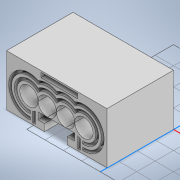
# Autodesk Inventor part: Part1
Saved by Autodesk Inventor 2020.3 (Build 243373010, 373A)
## iProperties
Created: 2021-11-04
Part Number: Part1
Material: Generic
Document SubType Name: Modeling
Designer: joesp
Density: 1 g/cm^3
Appearance: Default
Author: joesp
Autodesk Inventor part; units mm, degrees
ref_plane "YZ Plane" through (0, 0, 0) normal (1, 0, 0) x (0, 1, 0)
ref_plane "XZ Plane" through (0, 0, 0) normal (0, 1, 0) x (-1, 0, 0)
ref_plane "XY Plane" through (0, 0, 0) normal (0, 0, 1) x (1, 0, 0)
sketch "Sketch2" plane through (0, 0, 0) normal (0, 0, 1) x (1, 0, 0)
  line L0 (0, 0) -> (-109.5178, 0)
  line L1 (-109.5178, 0) -> (-109.5178, 55.7873)
  line L2 (-109.5178, 55.7873) -> (0, 55.7873)
  line L3 (0, 55.7873) -> (0, 0)
  circle A0 centre (-85.0707, 25.2343) radius 10
  circle A1 centre (-65.0707, 25.2343) radius 10
  circle A2 centre (-45.0707, 25.2343) radius 10
  circle A3 centre (-25.0707, 25.2343) radius 10
  line L4 (-71.9158, 54.2) -> (-31.9158, 54.2)
  line L5 (-31.9158, 54.2) -> (-31.9158, 49.2)
  line L6 (-31.9158, 49.2) -> (-71.9158, 49.2)
  line L7 (-71.9158, 49.2) -> (-71.9158, 54.2)
  line L8 (-68.1085, 0) -> (-68.1085, 7.7343)
  line L9 (-68.1085, 7.7343) -> (-75.0707, 7.7343)
  line L10 (-75.0707, 7.7343) -> (-75.0707, 15.2343)
  line L11 (-75.0707, 15.2343) -> (-35.0707, 15.2343)
  line L12 (-35.0707, 15.2343) -> (-35.0707, 7.7343)
  line L13 (-35.0707, 7.7343) -> (-43.2815, 7.7343)
  line L14 (-43.2815, 7.7343) -> (-43.2815, 0)
  arc A4 (-75.0707, 33.5409) -> (-76.764, 15.2343) centre (-85.0707, 25.2343) ccw
  arc A5 (-55.0707, 33.5409) -> (-75.0707, 33.5409) centre (-65.0707, 25.2343) ccw
  arc A6 (-35.0707, 33.5409) -> (-55.0707, 33.5409) centre (-45.0707, 25.2343) ccw
  arc A7 (-33.3773, 15.2343) -> (-35.0707, 33.5409) centre (-25.0707, 25.2343) ccw
  line L15 (-76.764, 15.2343) -> (-75.0707, 15.2343)
  line L16 (-33.3773, 15.2343) -> (-35.0707, 15.2343)
  arc A8 (-75.0707, 37.7243) -> (-81.0707, 9.7424) centre (-85.0707, 25.2343) ccw
  arc A9 (-55.0707, 37.7243) -> (-75.0707, 37.7243) centre (-65.0707, 25.2343) ccw
  arc A10 (-35.0707, 37.7243) -> (-55.0707, 37.7243) centre (-45.0707, 25.2343) ccw
  arc A11 (-29.0707, 9.7424) -> (-35.0707, 37.7243) centre (-25.0707, 25.2343) ccw
  line L17 (-78.0707, 2) -> (-81.0707, 2)
  line L18 (-81.0707, 2) -> (-81.0707, 14.2799)
  line L19 (-81.0707, 14.2799) -> (-78.0707, 14.2799)
  line L20 (-78.0707, 14.2799) -> (-78.0707, 2)
  line L21 (-83.5707, 12.3211) -> (-83.5707, 3.2855)
  line L22 (-32.0707, 14.2799) -> (-29.0707, 14.2799)
  line L23 (-29.0707, 14.2799) -> (-29.0707, 2)
  line L24 (-29.0707, 2) -> (-32.0707, 2)
  line L25 (-32.0707, 2) -> (-32.0707, 14.2799)
  line L26 (-26.5707, 12.8374) -> (-26.5707, 3.2855)
  arc A12 (-75.0707, 41.3898) -> (-81.0707, 6.6601) centre (-85.0707, 25.2343) ccw
  arc A13 (-55.0707, 41.3898) -> (-75.0707, 41.3898) centre (-65.0707, 25.2343) ccw
  arc A14 (-35.0707, 41.3898) -> (-55.0707, 41.3898) centre (-45.0707, 25.2343) ccw
  arc A15 (-29.0707, 6.6601) -> (-35.0707, 41.3898) centre (-25.0707, 25.2343) ccw
  arc A16 (-75.0707, 44.8302) -> (-81.0707, 3.601) centre (-85.0707, 25.2343) ccw
  arc A17 (-55.0707, 44.8302) -> (-75.0707, 44.8302) centre (-65.0707, 25.2343) ccw
  arc A18 (-35.0707, 44.8302) -> (-55.0707, 44.8302) centre (-45.0707, 25.2343) ccw
  arc A19 (-29.0707, 3.601) -> (-35.0707, 44.8302) centre (-25.0707, 25.2343) ccw
  point P0 (-75.0707, 25.2343)
  point P1 (-55.0707, 25.2343)
  point P2 (-35.0707, 25.2343)
  point P3 (-83.5707, 9.3048)
  point P4 (-26.5707, 9.3048)
  point P5 (-26.5707, 12.3211)
  point P6 (-29.0707, 12.865)
  point P7 (-81.0707, 12.865)
  point P8 (-65.0707, 15.2343)
  point P9 (-45.0707, 15.2343)
  point P10 (-83.5707, 6.2936)
  point P11 (-26.5707, 6.2936)
  dimension "d10" = 20
  dimension "d11" = 20
  dimension "d12" = 20
  dimension "d13" = 20
  dimension "d14" = 20
  dimension "d15" = 20
  dimension "d16" = 20
  dimension "d17" = 5
  dimension "d18" = 40
  dimension "d21" = 7.5
  dimension "d22" = 40
  dimension "d23" = 3
  dimension "d24" = 3
  dimension "d25" = 3
  dimension "d26" = 3
  dimension "d27" = 1.6934
  dimension "d28" = 1.6934
  dimension "d29" = 3
  dimension "d30" = 3
  dimension "d31" = 3
  dimension "d32" = 3
  dimension "d33" = 3
  dimension "d34" = 2
  dimension "d35" = 2.5
  dimension "d36" = 3
  dimension "d37" = 3
  dimension "d38" = 3
  dimension "d39" = 2
  dimension "d40" = 2.5
  dimension "d41" = 3
  dimension "d42" = 3
  dimension "d43" = 3
  dimension "d44" = 3
  dimension "d45" = 3
  dimension "d46" = 3
  dimension "d47" = 3
  dimension "d48" = 3
  constraints: 54 end point, 37 point on circle, 20 centre point, 16 coincident, 9 equal length, 9 perpendicular, 9 point on line, 6 horizontal, 3 horizontal alignment, 2 vertical, 1 tangent
  measures "d10" diameter of A0
  measures "d11" diameter of A1
  measures "d12" diameter of A2
  measures "d13" diameter of A3
  measures "d14" distance of A1.centre A0.centre
  measures "d15" distance of A2.centre A1.centre
  measures "d16" distance of A3.centre A2.centre
  measures "d17" distance of L6.end L4.start
  measures "d18" distance of L4.start L4.end
  measures "d21" distance of L9.end L10.end
  measures "d22" distance of L10.end L11.end
  measures "d23" radial gap between concentric circles of A1 A5
  measures "d24" radial gap between concentric circles of A2 A6
  measures "d25" radial gap between concentric circles of A7 A3
  measures "d26" radial gap between concentric circles of A4 A0
  measures "d27" distance of L16.start L11.end
  measures "d28" distance of L15.start L10.end
  measures "d29" radial gap between concentric circles of A11 A7
  measures "d30" radial gap between concentric circles of A8 A4
  measures "d31" radial gap between concentric circles of A9 A5
  measures "d32" radial gap between concentric circles of A10 A6
  measures "d33" distance between parallel lines of L10 L20
  measures "d34" distance between parallel lines of L0 L17
  measures "d35" distance between parallel lines of L18 L21
  measures "d36" distance of L18.end L19.end
  measures "d37" distance between parallel lines of L12 L25
  measures "d38" distance between parallel lines of L23 L25
  measures "d39" distance between parallel lines of L0 L24
  measures "d40" distance between parallel lines of L23 L26
  measures "d41" radial gap between concentric circles of A12 A8
  measures "d42" radial gap between concentric circles of A13 A9
  measures "d43" radial gap between concentric circles of A14 A10
  measures "d44" radial gap between concentric circles of A15 A11
  measures "d45" radial gap between concentric circles of A16 A12
  measures "d46" radial gap between concentric circles of A17 A13
  measures "d47" radial gap between concentric circles of A18 A14
  measures "d48" radial gap between concentric circles of A19 A15
extrude "Extrusion1" add sketch "Sketch2" along normal blind 72.5 contours L0 L14 L13 L12 L16 A7 L25 L24 L23 A19 A18 A17 A16 L18 L17 L20 A4 L15 L10 L9 L8 L1 L2 L3 | L11 A2 A1 L15 A4 L19 L18 A5 A6 A7 L23 L22 L16 | L11 A1 A2 | L22 L23 A7 | A4 L18 L19 | A7 L26 A11 L23 | L18 A8 L21 A4 | A11 L26 A15 L23 | L18 A12 L21 A8 | A11 A10 A9 A8 L21 A12 A13 A14 A15 L26 | A15 L26 A19 L23 | L18 A16 L21 A12
equation "\"d11\" = d10"
equation "\"d12\" = d10"
equation "\"d13\" = d10"
equation "\"d15\" = d14"
equation "\"d16\" = d14"
equation "\"d24\" = d23"
equation "\"d25\" = d23"
equation "\"d26\" = d23"
equation "\"d27\" = d28"
equation "\"d30\" = d29"
equation "\"d31\" = d29"
equation "\"d32\" = d29"
body "Solid1"
